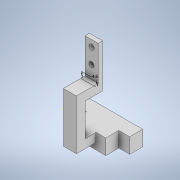
# Autodesk Inventor part: final522
Saved by Autodesk Inventor 2022 (Build 260153000, 153)
## iProperties
Created: 2023-05-22
Part Number: final522
Material: 일반
Document SubType Name: Modeling
Designer: HCI-TECH_KDK
Density: 1 g/cm^3
Appearance: 기본값
Author: HCI-TECH_KDK
Autodesk Inventor part; units mm, degrees
ref_plane "YZ Plane" through (0, 0, 0) normal (1, 0, 0) x (0, 1, 0)
ref_plane "XZ Plane" through (0, 0, 0) normal (0, 1, 0) x (-1, 0, 0)
ref_plane "XY Plane" through (0, 0, 0) normal (0, 0, 1) x (1, 0, 0)
sketch "스케치1" plane through (0, 0, 0) normal (0, 0, 1) x (1, 0, 0)
  line L0 (0, 0) -> (30, 0)
  line L1 (30, 0) -> (30, 20)
  line L2 (30, 20) -> (0, 20)
  line L3 (0, 20) -> (0, 0)
  line L4 (0, 20) -> (30, 20)
  line L5 (30, 20) -> (30, 17)
  line L6 (0, 17) -> (0, 20)
  line L7 (12, 20) -> (18, 20)
  line L8 (18, 20) -> (18, 16)
  line L9 (18, 16) -> (12, 16)
  line L10 (12, 16) -> (12, 20)
  point P0 (15, 20)
  point P1 (15, 20)
  dimension "d0" = 20
  dimension "d1" = 30
  dimension "d2" = 3
  dimension "d3" = 6
  dimension "d4" = 4
  constraints: 22 end point, 5 parallel, 3 horizontal, 3 perpendicular, 2 midpoint, 2 point on line, 1 coincident
  measures "d0" distance of L2.end L0.start
  measures "d1" distance of L1.end L2.end
  measures "d2" distance of L4.end L5.end
  measures "d3" distance of L8.end L9.end
  measures "d4" distance of L7.end L8.end
extrude "돌출1" add sketch "스케치1" along normal blind 10 contours L2 L8 L9 L10
sketch "스케치2" plane through (0, 0, 10) normal (0, 0, 1) x (1, 0, 0)
  line L0 (18, 20) -> (12, 20) projected
  line L1 (12, 20) -> (18, 20)
  line L2 (18, 20) -> (18, -3)
  line L3 (18, -3) -> (12, -3)
  line L4 (12, -3) -> (12, 20)
  point P0 (0, 0)
  dimension "d23" = 23
  constraints: 8 end point, 2 parallel, 1 horizontal, 1 perpendicular
  measures "d23" distance of L3.end L0.end
extrude "돌출2" add sketch "스케치2" along normal blind 4
sketch "스케치3" plane through (0, 0, 10) normal (0, 0, -1) x (-1, 0, 0)
  line L0 (-18, -3) -> (-18, 16) projected
  line L1 (-12, 16) -> (-12, -3) projected
  line L2 (-18, -3) -> (-12, -3)
  line L3 (-12, -3) -> (-12, 1)
  line L4 (-12, 1) -> (-18, 1)
  line L5 (-18, 1) -> (-18, -3)
  point P0 (0, 0)
  dimension "d9" = 4
  constraints: 8 end point, 2 parallel, 1 horizontal, 1 perpendicular, 1 point on line
  measures "d9" distance of L3.end L2.end
extrude "돌출3" add sketch "스케치3" along normal blind 15
sketch "스케치6" plane through (0, 0, 0) normal (0, 0, -1) x (-1, 0, 0)
  line L0 (-18, 16) -> (-18, 20) projected
  line L1 (-12, 16) -> (-18, 16) projected
  line L2 (-12, 20) -> (-12, 16) projected
  line L3 (-18, 20) -> (-12, 20) projected
  line L4 (-18, 16) -> (-18, 20) projected
  line L5 (-18, 16) -> (-12, 16)
  line L6 (-12, 16) -> (-12, 36)
  line L7 (-12, 36) -> (-18, 36)
  line L8 (-18, 36) -> (-18, 16)
  point P0 (0, 0)
  dimension "d20" = 20
  constraints: 8 end point, 2 parallel, 1 horizontal, 1 perpendicular
  measures "d20" distance of L6.end L5.end
extrude "돌출6" add sketch "스케치6" against normal blind 4 contours L8 L7 L6 L3
sketch "스케치7" plane through (12, 1, 10) normal (0, 1, 0) x (1, 0, 0)
  line L0 (6, 0) -> (0, 0) projected
  line L1 (6, 0) -> (6, 15) projected
  line L2 (0, 15) -> (6, 15) projected
  line L3 (0, 0) -> (0, 15) projected
  line L4 (-4.5, 15) -> (10.5, 15)
  line L5 (10.5, 15) -> (10.5, 10)
  line L6 (10.5, 10) -> (-4.5, 10)
  line L7 (-4.5, 10) -> (-4.5, 15)
  point P0 (-12, 10)
  point P1 (3, 15)
  point P2 (3, 15)
  point P3 (6, 15)
  point P4 (6, 10)
  point P5 (0, 10)
  dimension "d27" = 15
  constraints: 8 end point, 2 midpoint, 2 parallel, 1 coincident, 1 horizontal, 1 perpendicular
  measures "d27" distance of L4.start L4.end
extrude "돌출7" add sketch "스케치7" against normal blind 4 contours L1 L4 L5 L6 | L6 L7 L4 L3
sketch "스케치8" plane through (0, 0, -5) normal (0, 0, -1) x (-1, 0, 0)
  line L0 (-22.5, 1) -> (-7.5, 1) projected
  line L1 (-22.5, 1) -> (-22.5, -3) projected
  line L2 (-7.5, -3) -> (-22.5, -3) projected
  line L3 (-7.5, 1) -> (-7.5, -3) projected
  line L4 (-22.5, 1) -> (-7.5, 1)
  line L5 (-7.5, 1) -> (-7.5, -6)
  line L6 (-7.5, -6) -> (-22.5, -6)
  line L7 (-22.5, -6) -> (-22.5, 1)
  point P0 (0, 0)
  dimension "d28" = 7
  constraints: 8 end point, 2 parallel, 1 horizontal, 1 perpendicular
  measures "d28" distance of L4.end L5.end
extrude "돌출8" add sketch "스케치8" against normal blind 10
sketch "스케치9" plane through (0, 0, -5) normal (0, 0, -1) x (-1, 0, 0)
  line L0 (-20.1, 0.5) -> (-9.9, 0.5)
  line L1 (-9.9, 0.5) -> (-9.9, -4.5)
  line L2 (-9.9, -4.5) -> (-20.1, -4.5)
  line L3 (-20.1, -4.5) -> (-20.1, 0.5)
  line L4 (-22.5, 1) -> (-7.5, 1) projected
  line L5 (-22.5, 1) -> (-22.5, -6) projected
  point P0 (0, 0)
  point P1 (-15, 1)
  point P2 (-15, 0.5)
  dimension "d31" = 10.2
  dimension "d32" = 5
  dimension "d33" = 0.5
  constraints: 8 end point, 2 midpoint, 2 parallel, 1 horizontal, 1 perpendicular, 1 vertical alignment
  measures "d31" distance of L1.end L2.end
  measures "d32" distance of L0.end L1.end
  measures "d33" distance between parallel lines of L4 L0
extrude "돌출9" cut sketch "스케치9" against normal blind 8
sketch "스케치10" plane through (0, 0, -5) normal (0, 0, -1) x (-1, 0, 0)
  line L0 (-9.9, 0.5) -> (-9.9, -4.5) projected
  line L1 (-9.9, -4.5) -> (-20.1, -4.5) projected
  line L2 (-20.1, -4.5) -> (-20.1, 0.5) projected
  line L3 (-20.1, 0.5) -> (-9.9, 0.5) projected
  line L4 (-22.5, 1) -> (-7.5, 1) projected
  line L5 (-22.5, 1) -> (-22.5, -6) projected
  line L6 (-22.5, -6) -> (-7.5, -6) projected
  line L7 (-7.5, 1) -> (-7.5, -6) projected
  point P0 (0, 0)
extrude "돌출10" add sketch "스케치10" along normal blind 2
sketch "스케치11" plane through (12, 1, 10) normal (0, 1, 0) x (1, 0, 0)
  line L0 (0, 0) -> (0, 5) projected
  line L1 (6, 0) -> (0, 0) projected
  line L2 (6, 0) -> (6, 5) projected
  line L3 (10.5, 5) -> (6, 5) projected
  line L4 (10.5, 5) -> (10.5, 17) projected
  line L5 (-4.5, 17) -> (10.5, 17) projected
  line L6 (-4.5, 17) -> (-4.5, 5) projected
  line L7 (0, 5) -> (-4.5, 5) projected
  line L8 (-9.5, 11) -> (15.5, 11)
  line L9 (15.5, 11) -> (15.5, 17)
  line L10 (15.5, 17) -> (-9.5, 17)
  line L11 (-9.5, 17) -> (-9.5, 11)
  line L12 (0, 5) -> (6, 5) projected
  point P0 (-12, 10)
  point P1 (3, 11)
  point P2 (3, 5)
  point P3 (10.5, 17)
  point P4 (10.5, 11)
  point P5 (-4.5, 11)
  dimension "d39" = 25
  dimension "d40" = 6
  constraints: 8 end point, 2 parallel, 1 horizontal, 1 midpoint, 1 perpendicular, 1 vertical alignment, 2 other
  measures "d39" distance of L9.end L10.end
  measures "d40" distance between parallel lines of L10 L8
extrude "돌출11" add sketch "스케치11" against normal blind 7 contours L8 L11 L10 L6 | L4 L10 L9 L8
sketch "스케치12" plane through (0, 0, 0) normal (0, 0, -1) x (-1, 0, 0)
  line L0 (-12, 16) -> (-12, 36) projected
  line L1 (-18, 16) -> (-18, 36) projected
  line L2 (-12, 16) -> (-18, 16) projected
  line L3 (-12, 16) -> (-12, 36) projected
  line L4 (-12, 36) -> (-18, 36) projected
  point P0 (0, 0)
extrude "돌출12" cut sketch "스케치12" against normal blind 2
sketch "스케치13" plane through (0, 0, 4) normal (0, 0, 1) x (1, 0, 0)
  line L0 (18, 20) -> (18, 36) projected
  line L1 (18, 36) -> (12, 36) projected
  line L2 (12, 36) -> (12, 20) projected
  line L3 (18, 20) -> (12, 20) projected
  circle A0 centre (15, 33) radius 1.2
  circle A1 centre (15, 26) radius 1.2
  point P0 (0, 0)
  point P1 (15, 36)
  dimension "d45" = 2.4
  dimension "d48" = 3
  dimension "d51" = 7
  constraints: 2 centre point, 1 midpoint, 1 vertical, 1 vertical alignment, 2 other
  measures "d45" diameter of A0
  measures "d48" distance of point (15, 36) A0.centre
  measures "d51" distance of A0.centre A1.centre
extrude "돌출13" cut sketch "스케치13" against normal blind 2 contours A0 | A1
sketch "스케치16" plane through (0, 0, 2) normal (0, 0, -1) x (-1, 0, 0)
  circle A0 centre (-15, 19) radius 2.3
  line L0 (-12, 16) -> (-18, 16) projected
  point P0 (0, 0)
  point P1 (-15, 16)
  dimension "d59" = 4.6
  dimension "d60" = 3
  constraints: 1 centre point, 1 midpoint, 1 vertical alignment
  measures "d59" diameter of A0
  measures "d60" distance of point (-15, 16) A0.centre
